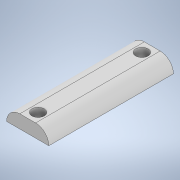
# Autodesk Inventor part: Festoon_LowerBracket
Saved by Autodesk Inventor 2022 (Build 260153000, 153)
## iProperties
Created: 2022-02-12
Part Number: Festoon_LowerBracket
Material: Generic
Document SubType Name: Modeling
Designer: locotacos99
Density: 1 g/cm^3
Appearance: Default
Author: locotacos99
Autodesk Inventor part; units mm, degrees
ref_plane "YZ Plane" through (0, 0, 0) normal (1, 0, 0) x (0, 1, 0)
ref_plane "XZ Plane" through (0, 0, 0) normal (0, 1, 0) x (-1, 0, 0)
ref_plane "XY Plane" through (0, 0, 0) normal (0, 0, 1) x (1, 0, 0)
sketch "Sketch1" plane through (0, 0, 0) normal (0, 0, 1) x (1, 0, 0)
  line L0 (-10.16, 3.175) -> (10.16, 3.175)
  line L1 (10.16, 3.175) -> (10.16, -3.175)
  line L2 (10.16, -3.175) -> (-10.16, -3.175)
  line L3 (-10.16, -3.175) -> (-10.16, 3.175)
  line L4 (-10.16, 3.175) -> (10.16, -3.175) construction
  line L5 (10.16, 3.175) -> (-10.16, -3.175) construction
  point P0 (0, 0)
  dimension "d0" = 20.32
  dimension "d1" = 6.35
  constraints: 12 end point, 2 midpoint, 2 parallel, 1 horizontal, 1 perpendicular
  measures "d0" distance of L1.end L2.end
  measures "d1" distance of L0.end L1.end
extrude "Extrusion1" add sketch "Sketch1" along normal blind 60
fillet "Fillet1" radius 6.35 2 edges at (-10.16, 3.175, 30) (10.16, 3.175, 30)
sketch "Sketch2" plane through (-3.81, 3.175, 0) normal (0, 1, 0) x (1, 0, 0)
  circle A0 centre (3.81, -5) radius 3
  line L0 (7.62, 0) -> (7.62, -60) projected
  circle A1 centre (3.81, -55) radius 3
  line L1 (7.62, -60) -> (0, -60) projected
  point P0 (3.81, 0)
  dimension "d5" = 6
  dimension "d6" = 5
  dimension "d7" = 3.81
  dimension "d10" = 6
  dimension "d11" = 3.81
  dimension "d15" = 50
  constraints: 2 centre point
  measures "d5" diameter of A0
  measures "d6" distance of A0.centre point (3.81, 0)
  measures "d7" distance from line of L0 A0.centre
  measures "d10" diameter of A1
  measures "d11" distance from line of L0 A1.centre
  measures "d15" distance of A0.centre A1.centre
extrude "Extrusion3" cut sketch "Sketch2" against normal through all
body "Solid1"
